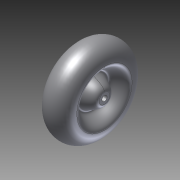
# Autodesk Inventor part: Wheel
Saved by Autodesk Inventor 2012 (Build 160160000, 160)
## iProperties
Created: 2011-10-20
Part Number: Wheel
Material: Rubber
Document SubType Name: Modeling
Designer: robotics
Density: 0.93 g/cm^3
Mass: 1508.3 g
Surface Area: 1052.74 cm^2
Volume: 1621.83 cm^3
GlobalPropertyList: <PropertyList/>
Author: robotics
Autodesk Inventor part; units mm, degrees
ref_plane "YZ Plane" through (0, 0, 0) normal (1, 0, 0) x (0, 1, 0)
ref_plane "XZ Plane" through (0, 0, 0) normal (0, 1, 0) x (-1, 0, 0)
ref_plane "XY Plane" through (0, 0, 0) normal (0, 0, 1) x (1, 0, 0)
sketch "Sketch1" plane through (0, 0, 0) normal (0, 0, 1) x (1, 0, 0)
  line L0 (34.925, 0) -> (34.925, 12.7)
  arc A0 (34.925, 66.675) -> (0, 101.6) centre (0, 66.675) ccw
  line L1 (0, 66.675) -> (34.925, 66.675) construction
  spline S0 degree 4 poles (34.925, 66.675) (34.925, 43.827) (-41.3043, 36.2486) (34.925, 35.3377) (34.925, 12.7) knots 0 0 0 0 0 1 1 1 1 1
  line L2 (34.925, 0) -> (0, 0)
  line L3 (0, 101.6) -> (0, 0)
  point P0 (6.35, 38.1)
  dimension "d0" = 34.925
  dimension "d2" = 12.7
  dimension "d5" = 101.6
  dimension "d7" = 34.925
  dimension "d8" = 6.35
  dimension "d9" = 38.1
  dimension "d10" = 53.975
  constraints: 8 end point, 2 point on circle, 2 vertical, 2 vertical alignment, 1 centre point, 1 horizontal alignment, 4 other
  measures "d0" distance of L0.start L2.end
  measures "d2" distance of L0.start L0.end
  measures "d5" distance of L2.end L3.start
  measures "d7" distance of L1.end L1.start
  measures "d8" horizontal distance of L2.end point (6.35, 38.1)
  measures "d9" vertical distance of L2.end point (6.35, 38.1)
  measures "d10" distance of L0.end L1.end
revolve "Revolution1" add sketch "Sketch1" angle 360 about axis through (34.925, 0, 0) along (-1, 0, 0)
mirror "Mirror1" about plane through (0, 50.8, 0) normal (-1, 0, 0) of "Revolution1"
sketch "Sketch2" plane through (34.925, 0, 0) normal (1, 0, 0) x (0, 0, -1)
  circle A0 centre (0, 0) radius 12.7 projected
  circle A1 centre (0, 0) radius 6.35
  point P0 (0, 12.7)
  dimension "d12" = 12.7
  constraints: 1 centre point, 1 coincident, 1 vertical alignment
  measures "d12" diameter of A1
extrude "Extrusion1" cut sketch "Sketch2" against normal through all contours A1
body "Solid1"
